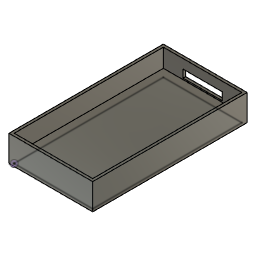
Case+tarjeta+1 (Autodesk Fusion 360 design; units mm, degrees)
Autodesk Fusion 360 part; units mm, degrees
sketch "Boceto1" plane through (0, 0, 0) normal (0, 0, 1) x (1, 0, 0)
  line L0 (0, 0) -> (30, 0)
  line L1 (30, 0) -> (30, 57)
  line L2 (30, 57) -> (0, 57)
  line L3 (0, 57) -> (0, 0)
  dimension "d1" = 57
  dimension "d2" = 30
  constraint horizontal L0
  constraint vertical L1
  constraint horizontal L2
  constraint vertical L3
  constraint coincident L0.start L3.end
  measures "d1" distance of L0.end L1.end
  measures "d2" distance of L1.end L2.end
extrude "Extruir1" add sketch "Boceto1" along normal blind 3
sketch "Boceto2" plane through (0, 0, 0) normal (0, 0, -1) x (1, 0, 0)
  line L0 (0, 0) -> (0, -57)
  line L1 (0, -57) -> (30, -57)
  line L2 (30, -57) -> (30, 0)
  line L3 (30, 0) -> (0, 0)
extrude "Extruir2" add sketch "Boceto2" against normal blind 10 thin wall 1 outside
sketch "Boceto3" plane through (0, 58, 0) normal (0, 1, 0) x (-1, 0, 0)
  line L0 (-31, 0) -> (1, 0)
  line L1 (1, 0) -> (1, 10)
  line L2 (1, 10) -> (-31, 10)
  line L3 (-31, 10) -> (-31, 0)
  line L4 (-22.5, 6.5) -> (-7.5, 6.5)
  line L5 (-7.5, 6.5) -> (-7.5, 3.5)
  line L6 (-7.5, 3.5) -> (-22.5, 3.5)
  line L7 (-22.5, 3.5) -> (-22.5, 6.5)
  point P0 (-15, 3.5)
  point P1 (-15, 0)
  point P2 (-7.5, 5)
  point P3 (1, 5)
  dimension "d8" = 15
  dimension "d9" = 3
  constraint horizontal L4
  constraint vertical L5
  constraint horizontal L6
  constraint vertical L7
  constraint midpoint L6 P0
  constraint midpoint L0 P1
  constraint vertical P0 P1
  constraint midpoint L5 P2
  constraint midpoint L1 P3
  constraint horizontal P2 P3
  measures "d8" distance of L4.start L4.end
  measures "d9" distance of L4.end L5.end
extrude "Extruir3" cut sketch "Boceto3" against normal up to surface (1 mm away) contours L4 L5 L6 L7
